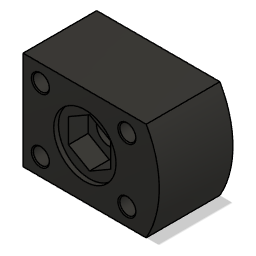
side brace lwr mount nut insert v4 (Autodesk Fusion 360 design; units mm, degrees)
Autodesk Fusion 360 part; units mm, degrees
sketch "Sketch1" plane through (0, 0, 0) normal (0, 0, 1) x (1, 0, 0)
  circle A0 centre (0, 0) radius 12.6
  line L0 (-25, 19.9) -> (-25, -19.9)
  line L1 (-25, 19.9) -> (24.8138, 19.9)
  line L2 (-25, -19.9) -> (24.8138, -19.9)
  circle A1 centre (0, 0) radius 5.25
  arc A2 (24.8138, -19.9) -> (24.8138, 19.9) centre (-10, 0) ccw
  line L3 (0, 0) -> (-10, 0) construction
  line L4 (8.55, 4.9363) -> (0, 9.8727)
  line L5 (0, 9.8727) -> (-8.55, 4.9363)
  line L6 (-8.55, 4.9363) -> (-8.55, -4.9363)
  line L7 (-8.55, -4.9363) -> (0, -9.8727)
  line L8 (0, -9.8727) -> (8.55, -4.9363)
  line L9 (8.55, -4.9363) -> (8.55, 4.9363)
  circle A3 centre (-18, 12.9) radius 3.25
  circle A4 centre (-18, -12.9) radius 3.25
  circle A5 centre (17, -12.9) radius 3.25
  circle A6 centre (17, 12.9) radius 3.25
  line L10 (-18, 12.9) -> (17, 12.9) construction
  line L11 (17, 12.9) -> (17, -12.9) construction
  line L12 (17, -12.9) -> (-18, -12.9) construction
  dimension "d1" = 25.2
  dimension "d3" = 19.9
  dimension "d4" = 19.9
  dimension "d7" = 10.5
  dimension "d8" = 40.1
  dimension "d10" = 17.1
  dimension "d19" = 7
  dimension "d20" = 6.5
  dimension "d22" = 7
  dimension "d23" = 35
  dimension "d28" = 18
  dimension "d29" = 10
  dimension "d30" = 25
  constraint coincident A0.centre A1.centre
  constraint vertical L0
  constraint perpendicular L0 L1
  constraint perpendicular L0 L2
  constraint coincident A2.centre L3.end
  constraint horizontal L3
  constraint vertical L9
  constraint coincident A3.centre L10.start
  constraint coincident A6.centre L10.end
  constraint coincident A5.centre L11.end
  constraint coincident A4.centre L12.end
  constraint perpendicular L10 L11
  constraint perpendicular L11 L12
  constraint horizontal L10
  constraint equal A3 A6
  constraint equal A5 A6
  constraint equal A4 A5
  constraint equal L10 L12
  measures "d1" diameter of A0
  measures "d3" vertical distance of A0.centre L0.start
  measures "d4" vertical distance of A0.centre L0.end
  measures "d7" diameter of A1
  measures "d8" radius of A2
  measures "d10" distance of L6 L9
  measures "d19" distance of L1 A3.centre
  measures "d20" diameter of A3
  measures "d22" distance of L2 A4.centre
  measures "d23" distance of A3.centre A6.centre
  measures "d28" horizontal distance of A0.centre A3.centre
  measures "d29" distance of A0.centre A2.centre
  measures "d30" distance of L0 A0.centre
extrude "Extrude1" add sketch "Sketch1" along normal mid plane 29.8 contours L0 L1 L2 A2 makes body 1
extrude "Extrude3" add sketch "Sketch1" along normal mid plane 26 contours A0 bodies 1
extrude "Extrude4" add sketch "Sketch1" along normal mid plane 10 contours L4 L5 L6 L7 L8 L9 bodies 1
extrude "Extrude5" add sketch "Sketch1" along normal blind 5 and the other way blind 0 contours A3 | A4 | A5 | A6 bodies 1
copy_body "Body->Comp1" bodies 1 removing the originals makes body 2 in component "side brace lwr mount nut insert"
chamfer "Chamfer1" distance 0.4 angle 45 8 edges at (13.9699, 14.0753, 14.9) (-21.0301, 14.0753, 14.9) (-21.0301, -11.7247, 14.9) (13.9699, -11.7247, 14.9) (13.9699, -14.0753, -14.9) (-21.0301, 11.7247, -14.9) (13.9699, 11.7247, -14.9) (-21.0301, -14.0753, -14.9) on bodies 2 in component "side brace lwr mount nut insert"
component "side brace lwr mount nut insert" placed x (1, 0, 0) y (0, 1, 0) z (0, 0, 1) at (0, 0, 0)
equation "d4 = d3"
named bodies: "side brace lwr mount nut insert"
